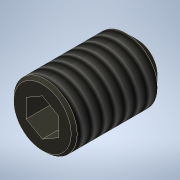
# Autodesk Inventor part: SCREW,SET,CUP POINT,M4X0.7X6MM
Saved by Autodesk Inventor 2022.4 (Build 264492000, 492)
## iProperties
Category: _
Manager: 612-20220
Created: 2018-08-02
Part Number: SCREW,SET,CUP POINT,M4X0.7X6MM
Checked By: 0002270779
Engr Approved By: P
User Status: Released
Material: Steel, MS
Description: SCREW,SET,CUP POINT,M4X0.7X6MM
Document SubType Name: Modeling
Mfg Approved By: Cathy.Lesperance
Designer: Clint.Matte
Manufacturer: Standard
Standards Organization: Custom
Density: 7.86 g/cm^3
Appearance: Gunmetal
Mass: 0.485777 g
Surface Area: 1.11388 cm^2
Volume: 0.0618037 cm^3
CN_MASS: 0.000486
CN_SERVICEABLE: _
FIRST_DESCRIPTION: M4-0.7 X 6MM
SECOND_DESCRIPTION: CUP POINT  - STEEL
THIRD_DESCRIPTION: _
PTC_WM_ITERATION: 1
PTC_WM_ORGANIZATION_ID: CLWC
PTC_WM_LIFECYCLE: CLWC_CAD_LC
CL_runCount: 1
FinishProperty: ToBeSet
Subject: 40828
Author: -
Keywords: FASTENAL
Revision Number: A
Title: SetScrewCup M4x0.7x6
Autodesk Inventor part; units mm, degrees
ref_plane "YZ Plane" through (0, 0, 0) normal (1, 0, 0) x (0, 1, 0)
ref_plane "XZ Plane" through (0, 0, 0) normal (0, 1, 0) x (-1, 0, 0)
ref_plane "XY Plane" through (0, 0, 0) normal (0, 0, 1) x (1, 0, 0)
sketch "Sketch3" plane through (0, 0, 0) normal (0, 0, 1) x (1, 0, 0)
  circle A0 centre (0, 0) radius 2 projected
  line L0 (1.0225, 0.5903) -> (1.0225, -0.5903)
  line L1 (1.0225, -0.5903) -> (0, -1.1807)
  line L2 (0, -1.1807) -> (-1.0225, -0.5903)
  line L3 (-1.0225, -0.5903) -> (-1.0225, 0.5903)
  line L4 (-1.0225, 0.5903) -> (0, 1.1807)
  line L5 (0, 1.1807) -> (1.0225, 0.5903)
  line L6 (0, 0) -> (0, 1.1807) construction
  dimension "HexWidth" = 2.045
  constraints: 14 end point, 1 coincident, 1 vertical, 13 other
  measures "HexWidth" distance between parallel lines of L0 L3
sketch "Sketch2" plane through (0, 0, 0) normal (0, 0, 1) x (1, 0, 0)
  circle A0 centre (0, 0) radius 2
  dimension "Diam" = 4
  constraints: 1 centre point, 1 coincident
  measures "Diam" diameter of A0
extrude "Extrusion2" add sketch "Sketch2" against normal blind 6
thread "Thread1" size "M4x0.7" class "6g" standard "ANSI Metric M Profile" full length
extrude "Extrusion3" cut sketch "Sketch3" against normal blind 2.5 contours L0 L1 L2 L3 L4 L5
chamfer "Chamfer2" distance 0.75 angle 45 1 edges at (-2, 0, -6)
chamfer "Chamfer3" distance 0.1875 angle 45 1 edges at (-2, 0, 0)
sketch "Sketch4" plane through (0, 0, -6) normal (0, 0, -1) x (-1, 0, 0)
  circle A0 centre (0, 0) radius 1.8125 projected
  constraints: 1 coincident
hole "Cup_Point_Hole1" at (0, 0, -6) direction (0, 0, 1) diameter 2.4999 depth 0.001 tip angle 118
equation "\"d8\" = -0.5 * CupPointDiam + 0.5 * Diam"
equation "\"d11\" = 0.25 * d8"
equation "\"CupPointDiam\" = 2.5"
body "Solid1"
